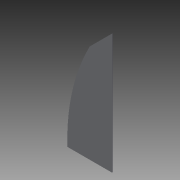
# Autodesk Inventor part: Solar Cell
Saved by Autodesk Inventor 2015 SP1 (Build 190203100, 203)
## iProperties
Created: 2015-06-22
Part Number: Solar Cell
Material: Generic
Document SubType Name: Modeling
Designer: Kartikye
Density: 1 g/cm^3
Appearance: Default
Author: Kartikye
Autodesk Inventor part; units mm, degrees
ref_plane "YZ Plane" through (0, 0, 0) normal (1, 0, 0) x (0, 1, 0)
ref_plane "XZ Plane" through (0, 0, 0) normal (0, 1, 0) x (-1, 0, 0)
ref_plane "XY Plane" through (0, 0, 0) normal (0, 0, 1) x (1, 0, 0)
sketch "Sketch1" plane through (0, 0, 0) normal (0, 1, 0) x (-1, 0, 0)
  line L0 (-4.7329, 13.0804) -> (0.1578, 8.1946)
  arc A0 (5.0486, -13.3423) -> (0.1578, 8.1946) centre (-38.4524, -11.897) ccw
  line L1 (5.0486, -13.3423) -> (-4.7329, -13.3423)
  line L2 (-4.7329, 13.0804) -> (-4.7329, -13.3423)
  point P0 (0, 0)
  constraints: 6 end point, 2 point on circle, 1 centre point
extrude "Extrusion1" add sketch "Sketch1" along normal blind 0.16
sketch "Sketch2" plane through (0, 0.16, 0) normal (0, 1, 0) x (1, 0, 0)
  point P0 (0, 0)
body "Solid1"
